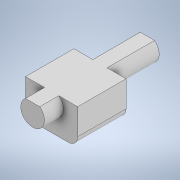
# Autodesk Inventor part: rpi_base_front
Saved by Autodesk Inventor 2022.1 (Build 261234000, 234)
## iProperties
Created: 2021-07-18
Part Number: rpi_base_front
Material: Generic
Document SubType Name: Modeling
Designer: dwbertol
Density: 1 g/cm^3
Appearance: Default
Author: dwbertol
## iProperties of the stored document rpi_base_front_3DPrint.ipt
Created: 2021-07-18
Part Number: rpi_base_front_3DPrint
Material: Generic
Document SubType Name: Modeling
Designer: dwbertol
Density: 1 g/cm^3
Appearance: Default
Author: dwbertol
Autodesk Inventor part; units mm, degrees
ref_plane "YZ Plane" through (0, 0, 0) normal (1, 0, 0) x (0, 1, 0)
ref_plane "XZ Plane" through (0, 0, 0) normal (0, 1, 0) x (-1, 0, 0)
ref_plane "XY Plane" through (0, 0, 0) normal (0, 0, 1) x (1, 0, 0)
sketch "Sketch1" plane through (0, 0, 0) normal (0, 0, 1) x (1, 0, 0)
  circle A0 centre (0, 0) radius 1.25
  circle A1 centre (0, 0) radius 2.75
  line L0 (-1.75, 2.75) -> (1.75, 2.75)
  line L1 (2.75, 1.75) -> (2.75, -1.75)
  line L2 (1.75, -2.75) -> (-1.75, -2.75)
  line L3 (-2.75, -1.75) -> (-2.75, 1.75)
  arc A2 (-1.75, 2.75) -> (-2.75, 1.75) centre (-1.75, 1.75) ccw
  arc A3 (2.75, 1.75) -> (1.75, 2.75) centre (1.75, 1.75) ccw
  arc A4 (1.75, -2.75) -> (2.75, -1.75) centre (1.75, -1.75) ccw
  arc A5 (-2.75, -1.75) -> (-1.75, -2.75) centre (-1.75, -1.75) ccw
  line L4 (-2.75, 1) -> (2.75, 1)
  point P0 (-2.75, 0)
  point P1 (0, -2.75)
  point P2 (0.75, 1)
  point P3 (-0.75, 1)
  dimension "d0" = 2.5
  dimension "d1" = 5.5
  dimension "d2" = 1
  dimension "d3" = 1
  dimension "d4" = 1
  dimension "d11" = 1
  constraints: 12 tangent, 10 end point, 8 point on circle, 6 centre point, 2 coincident, 2 parallel, 2 perpendicular, 2 point on line, 1 equal radius, 1 horizontal
  measures "d0" diameter of A0
  measures "d1" diameter of A1
  measures "d2" radius of A2
  measures "d3" radius of A3
  measures "d4" radius of A5
  measures "d11" distance from line of L4 point (0, 0)
extrude "Extrusion1" add sketch "Sketch1" against normal blind 5 contours A0 L4 picked at (0.7457, -0.3378)
extrude "Extrusion2" add sketch "Sketch1" along normal blind 5.1 contours A0 L4 | A0 L4 A1 | L4 L1 A1 | A1 L3 L4 | L1 A4 L2 A1 | A1 L2 A5 L3 picked at (0.7457, -0.3378) picked at (2.227, -0.204)
extrude "Extrusion3" add sketch "Sketch1" along normal blind 7.1 contours A0 L4 picked at (0.7457, -0.3378)
body "Solid1"
